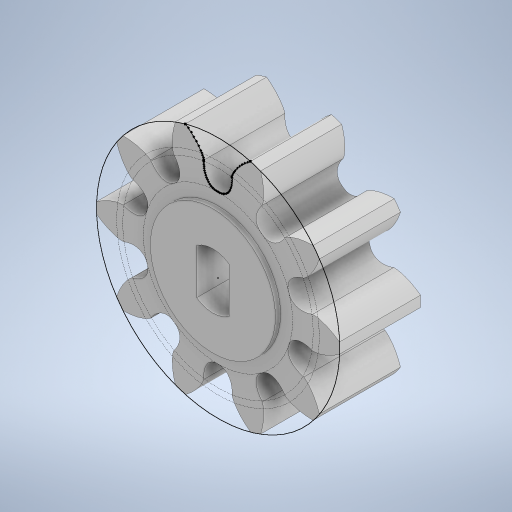
# Autodesk Inventor part: koloMale
Saved by Autodesk Inventor 2023 (Build 270158000, 158)
## iProperties
Created: 2023-11-20
Part Number: koloMale
Material: Generic
Document SubType Name: Modeling
Designer: alexa
Density: 1 g/cm^3
Appearance: Default
Author: alexa
Autodesk Inventor part; units mm, degrees
ref_plane "YZ Plane" through (0, 0, 0) normal (1, 0, 0) x (0, 1, 0)
ref_plane "XZ Plane" through (0, 0, 0) normal (0, 1, 0) x (-1, 0, 0)
ref_plane "XY Plane" through (0, 0, 0) normal (0, 0, 1) x (1, 0, 0)
sketch "Sketch1" plane through (0, 0, 0) normal (0, 0, 1) x (1, 0, 0)
  spline S0 degree 3 poles (-3.2061, 11.5638) (-3.1097, 11.4916) (-2.917, 11.3473) (-2.6424, 11.1124) (-2.3806, 10.8636) (-2.1344, 10.5991) (-1.9066, 10.3186) (-1.7352, 10.0709) (-1.6121, 9.8639) (-1.5286, 9.7038) (-1.4535, 9.5393) (-1.4166, 9.4247) (-1.3981, 9.3674) knots 0 0 0 0 0.036108 0.072216 0.108323 0.144429 0.180534 0.216635 0.23469 0.252743 0.270795 0.288843 0.288843 0.288843 0.288843
  spline S1 degree 3 poles (-1.3981, 9.3674) (-1.4013, 9.309) (-1.4076, 9.1922) (-1.4063, 9.0167) (-1.3951, 8.8416) (-1.3717, 8.6676) (-1.3393, 8.4951) (-1.2907, 8.3264) (-1.2306, 8.1614) (-1.1536, 8.0034) (-1.0602, 7.8546) (-0.9494, 7.7182) (-0.8216, 7.5973) (-0.6776, 7.4961) (-0.5193, 7.4193) (-0.3505, 7.3689) (-0.1754, 7.3497) (0, 7.3559) (0.1754, 7.3497) (0.3505, 7.3689) (0.5193, 7.4193) (0.6776, 7.4961) (0.8216, 7.5973) (0.9494, 7.7182) (1.0602, 7.8546) (1.1536, 8.0034) (1.2306, 8.1614) (1.2907, 8.3264) (1.3393, 8.4951) (1.3717, 8.6676) (1.3951, 8.8416) (1.4063, 9.0167) (1.4076, 9.1922) (1.4013, 9.309) (1.3981, 9.3674) knots 0 0 0 0 0.017541 0.03508 0.05262 0.07016 0.087698 0.105237 0.122773 0.140312 0.157847 0.175379 0.19291 0.210437 0.227965 0.245488 0.263009 0.28055 0.298092 0.315613 0.333136 0.350664 0.368191 0.385722 0.403254 0.420789 0.438328 0.455864 0.473403 0.490941 0.508481 0.526021 0.54356 0.561101 0.561101 0.561101 0.561101
  spline S2 degree 3 poles (1.3981, 9.3674) (1.4166, 9.4247) (1.4535, 9.5393) (1.5286, 9.7038) (1.6121, 9.8639) (1.7352, 10.0709) (1.9066, 10.3186) (2.1344, 10.5991) (2.3806, 10.8636) (2.6424, 11.1124) (2.917, 11.3473) (3.1097, 11.4916) (3.2061, 11.5638) knots 0 0 0 0 0.018047 0.036099 0.054153 0.072207 0.108309 0.144413 0.180519 0.216626 0.252734 0.288843 0.288843 0.288843 0.288843
  circle A0 centre (0, 0) radius 7.3538 construction
  circle A1 centre (0, 0) radius 9.3969 construction
  circle A2 centre (0, 0) radius 10 construction
  circle A3 centre (0, 0) radius 12
  point P0 (-2.9194, 11.3443)
  point P1 (-2.6445, 11.1101)
  point P2 (-2.3832, 10.861)
  point P3 (-2.1375, 10.5964)
  point P4 (-1.9103, 10.3158)
  point P5 (-1.7056, 10.0184)
  point P6 (-1.6136, 9.8631)
  point P7 (-1.53, 9.7031)
  point P8 (-1.4568, 9.5381)
  point P9 (-1.4058, 9.1922)
  point P10 (-1.4047, 9.0168)
  point P11 (-1.3931, 8.8418)
  point P12 (-1.3702, 8.6679)
  point P13 (-1.3366, 8.4957)
  point P14 (-1.2888, 8.327)
  point P15 (-1.2278, 8.1626)
  point P16 (-1.1509, 8.005)
  point P17 (-1.0573, 7.8567)
  point P18 (-0.9465, 7.7208)
  point P19 (-0.8189, 7.6006)
  point P20 (-0.6752, 7.5002)
  point P21 (-0.5175, 7.4237)
  point P22 (-0.3495, 7.3741)
  point P23 (-0.1754, 7.3539)
  point P24 (0, 7.3538)
  point P25 (0.1754, 7.3539)
  point P26 (0.3495, 7.3741)
  point P27 (0.5175, 7.4237)
  point P28 (0.6752, 7.5002)
  point P29 (0.8189, 7.6006)
  point P30 (0.9465, 7.7208)
  point P31 (1.0573, 7.8567)
  point P32 (1.1509, 8.005)
  point P33 (1.2278, 8.1626)
  point P34 (1.2888, 8.327)
  point P35 (1.3366, 8.4957)
  point P36 (1.3702, 8.6679)
  point P37 (1.3931, 8.8418)
  point P38 (1.4047, 9.0168)
  point P39 (1.4058, 9.1922)
  point P40 (1.4568, 9.5381)
  point P41 (1.53, 9.7031)
  point P42 (1.6136, 9.8631)
  point P43 (1.7056, 10.0184)
  point P44 (1.9103, 10.3158)
  point P45 (2.1375, 10.5964)
  point P46 (2.3832, 10.861)
  point P47 (2.6445, 11.1101)
  point P48 (2.9194, 11.3443)
  constraints: 4 centre point, 2 point on circle, 113 other
extrude "Extrusion1" add sketch "Sketch1" against normal blind 8
extrude "Extrusion2" cut sketch "Sketch1" against normal blind 10 contours A3 S2 S1 S0 picked at (0.3308, 10.4648)
pattern_circular "Circular Pattern1" count 10 over 360 about axis through (0, 0, -10) along (0, 0, 1) of "Extrusion2"
sketch "Sketch2" plane through (0, 0, 0) normal (0, 0, 1) x (1, 0, 0)
  circle A0 centre (0, 0) radius 2.75
  line L0 (1.6, -2.2366) -> (1.6, 2.2366)
  line L1 (-1.6, -2.2366) -> (-1.6, 2.2366)
  dimension "d7" = 5.5
  dimension "d10" = 3.2
  constraints: 4 end point, 4 point on circle, 2 vertical, 1 centre point, 1 coincident, 1 parallel
  measures "d7" diameter of A0
  measures "d10" distance between parallel lines of L0 L1
extrude "Extrusion3" cut sketch "Sketch2" against normal blind 10 contours L0 A0 L1
sketch "Sketch3" plane through (0, 0, 0) normal (0, 0, 1) x (1, 0, 0)
  circle A0 centre (0, 0) radius 6.1757
  line L0 (1.6, 2.2366) -> (1.6, -2.2366) projected
  arc A1 (-1.6, -2.2366) -> (1.6, -2.2366) centre (0, 0) ccw projected
  line L1 (-1.6, -2.2366) -> (-1.6, 2.2366) projected
  arc A2 (1.6, 2.2366) -> (-1.6, 2.2366) centre (0, 0) ccw projected
  arc A3 (4.2032, 11.2398) -> (3.2061, 11.5638) centre (0, 0) ccw projected
  arc A4 (-3.2061, 11.5638) -> (-4.2032, 11.2398) centre (0, 0) ccw projected
  arc A5 (-9.3908, 7.4708) -> (-10.0071, 6.6226) centre (0, 0) ccw projected
  arc A6 (-11.9885, 0.5242) -> (-11.9885, -0.5242) centre (0, 0) ccw projected
  arc A7 (-10.0071, -6.6226) -> (-9.3908, -7.4708) centre (0, 0) ccw projected
  arc A8 (-4.2032, -11.2398) -> (-3.2061, -11.5638) centre (0, 0) ccw projected
  arc A9 (3.2061, -11.5638) -> (4.2032, -11.2398) centre (0, 0) ccw projected
  arc A10 (9.3908, -7.4708) -> (10.0071, -6.6226) centre (0, 0) ccw projected
  arc A11 (11.9885, -0.5242) -> (11.9885, 0.5242) centre (0, 0) ccw projected
  arc A12 (10.0071, 6.6226) -> (9.3908, 7.4708) centre (0, 0) ccw projected
  point P0 (6.6371, 6.7566)
  point P1 (4.375, 8.4002)
  point P2 (1.3981, 9.3674)
  point P3 (-1.3981, 9.3674)
  point P4 (-4.375, 8.4002)
  point P5 (-6.6371, 6.7566)
  point P6 (-8.4769, 4.2243)
  point P7 (-9.341, 1.565)
  point P8 (-9.341, -1.565)
  point P9 (-8.4769, -4.2243)
  point P10 (-6.6371, -6.7566)
  point P11 (-4.375, -8.4002)
  point P12 (-1.3981, -9.3674)
  point P13 (1.3981, -9.3674)
  point P14 (4.375, -8.4002)
  point P15 (6.6371, -6.7566)
  point P16 (8.4769, -4.2243)
  point P17 (9.341, -1.565)
  point P18 (9.341, 1.565)
  point P19 (8.4769, 4.2243)
  constraints: 2 horizontal alignment, 1 centre point, 1 coincident, 28 other
extrude "Extrusion4" add sketch "Sketch3" along normal blind 0.5
equation "\"d0\" = FaceWidth"
equation "\"Module\" = 2"
equation "\"PressureAngle\" = 20deg"
equation "\"UnitProfileClearance\" = 0.25"
equation "\"UnitRoundRadius\" = 0.35"
equation "\"HeadDiameter\" = 24"
equation "\"RootDiameter\" = 14.70762"
equation "\"BaseDiameter\" = 18.79385"
equation "\"FaceWidth\" = 8"
equation "\"HelixAngle\" = 0"
equation "\"UnitCorrection\" = 0"
equation "\"UnitAddendumModification\" = 0"
equation "\"CircularPitch\" = 6.283185"
equation "\"UnitBacklashShift\" = -0.073095"
equation "\"TotalToolShift\" = -0.14619"
equation "\"IsInternal\" = 0"
body "Solid1"
